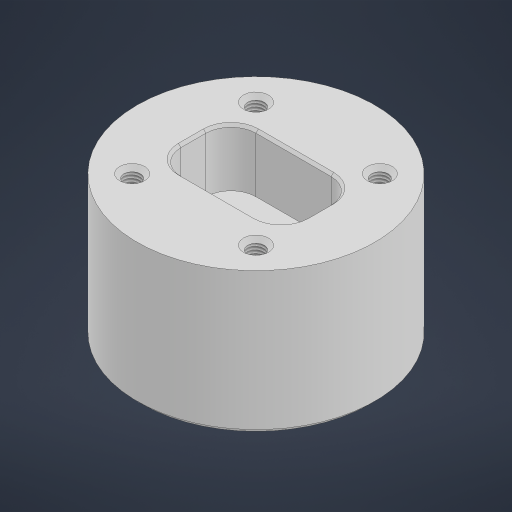
# Autodesk Inventor part: HM1_FIXT1-001
Saved by Autodesk Inventor 2024.3 (Build 283343000, 343)
## iProperties
Created: 2024-08-19
Part Number: HM1_FIXT1-001
Material: Generic
Document SubType Name: Modeling
Designer: fablabadmin
Density: 1 g/cm^3
Appearance: Default
Author: fablabadmin
Autodesk Inventor part; units mm, degrees
ref_plane "YZ Plane" through (0, 0, 0) normal (1, 0, 0) x (0, 1, 0)
ref_plane "XZ Plane" through (0, 0, 0) normal (0, 1, 0) x (-1, 0, 0)
ref_plane "XY Plane" through (0, 0, 0) normal (0, 0, 1) x (1, 0, 0)
sketch "Sketch1" plane through (0, 0, 0) normal (0, 1, 0) x (-1, 0, 0)
  circle A0 centre (0, 0) radius 47.5
  line L0 (-15, 15) -> (15, 15)
  line L1 (25, 5) -> (25, -5)
  line L2 (15, -15) -> (-15, -15)
  line L3 (-25, -5) -> (-25, 5)
  line L4 (-25, 15) -> (25, -15) construction
  line L5 (25, 15) -> (-25, -15) construction
  line L6 (-24.7487, 24.7487) -> (24.7487, 24.7487) construction
  line L7 (24.7487, 24.7487) -> (24.7487, -24.7487) construction
  line L8 (24.7487, -24.7487) -> (-24.7487, -24.7487) construction
  line L9 (-24.7487, -24.7487) -> (-24.7487, 24.7487) construction
  line L10 (-24.7487, 24.7487) -> (24.7487, -24.7487) construction
  line L11 (24.7487, 24.7487) -> (-24.7487, -24.7487) construction
  circle A1 centre (0, 0) radius 35 construction
  arc A2 (15, -15) -> (25, -5) centre (15, -5) ccw
  arc A3 (-25, -5) -> (-15, -15) centre (-15, -5) ccw
  arc A4 (-15, 15) -> (-25, 5) centre (-15, 5) ccw
  arc A5 (25, 5) -> (15, 15) centre (15, 5) ccw
  dimension "d25" = 70
  dimension "d0" = 30
  dimension "d1" = 50
  dimension "d2" = 95
  dimension "d4" = 12.5
  dimension "d16" = 10
  constraints: 24 end point, 8 point on circle, 8 point on line, 8 tangent, 6 coincident, 5 centre point, 4 midpoint, 4 parallel, 3 equal radius, 3 perpendicular, 2 horizontal, 3 other
  measures "d0" distance of L5.end L4.start
  measures "d1" distance of L4.end L5.end
  measures "d2" diameter of A0
  measures "d16" radius of A2
extrude "Extrusion1" add sketch "Sketch1" against normal blind 57 contours A0 | L0 A5 L1 A2 L2 A3 L3 A4
extrude "Extrusion2" cut sketch "Sketch1" against normal blind 23 contours L0 A5 L1 A2 L2 A3 L3 A4
hole "Hole1" at (-24.7487, 0, -24.7487) at (24.7487, 0, -24.7487) at (24.7487, 0, 24.7487) at (-24.7487, 0, 24.7487) direction (0, -1, 0) diameter 6.647 depth 20.4 tip angle 118 countersink diameter 10 countersink angle 90 thread size "M8x1.25" class "6H" standard "ISO Metric profile"
chamfer "Chamfer1" distance 1 angle 45 8 edges at (0, 0, -15) (22.0711, 0, -12.0711) (25, 0, 0) (22.0711, 0, 12.0711) (0, 0, 15) (-22.0711, 0, 12.0711) (-25, 0, 0) (-22.0711, 0, -12.0711)
chamfer "Chamfer2" distance 2 angle 45 1 edges at (47.5, -57, 0)
sketch "Sketch2" plane through (0, -57, 0) normal (0, -1, 0) x (1, 0, 0)
  circle A0 centre (0, 0) radius 20 construction
  circle A1 centre (0, 0) radius 24 construction
  dimension "d23" = 4
  dimension "d24" = 40
  constraints: 2 centre point, 2 coincident, 2 other
  measures "d23" radial gap between concentric circles of A0 A1
  measures "d24" diameter of A0
mark "Mark1"
body "Solid1"
